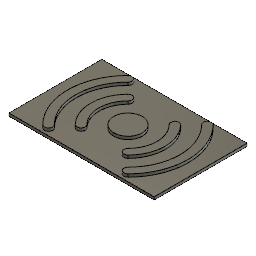
Glas (Autodesk Fusion 360 design; units mm, degrees)
Autodesk Fusion 360 part; units mm, degrees
sketch "Skizze1" plane through (0, 0, 0) normal (0, 1, 0) x (1, 0, 0)
  line L0 (25, 16) -> (-25, 16)
  line L1 (-25, 16) -> (-25, -16)
  line L2 (-25, -16) -> (25, -16)
  line L3 (25, -16) -> (25, 16)
  line L4 (25, 16) -> (-25, -16) construction
  line L5 (-25, 16) -> (25, -16) construction
  dimension "d1" = 50
  dimension "d2" = 32
  constraint horizontal L0
  constraint perpendicular L0 L1
  constraint parallel L0 L2
  constraint parallel L1 L3
  measures "d1" distance of L1.end L2.end
  measures "d2" distance of L0.end L1.end
extrude "Extrusion1" add sketch "Skizze1" along normal blind 1
sketch "Skizze2" plane through (0, 1, 0) normal (0, 1, 0) x (-1, 0, 0)
  line L0 (-25, 16) -> (-25, -16)
  line L1 (-25, -16) -> (25, -16)
  line L2 (25, -16) -> (25, 16)
  line L3 (25, 16) -> (-25, 16)
  circle A0 centre (0, 0) radius 4.9
  line L4 (0, 0) -> (0, -16) construction
  line L5 (0, 0) -> (-14.6371, -14.6371) construction
  line L6 (0, 0) -> (-14.6371, 14.6371) construction
  arc A1 (-7.0711, 7.0711) -> (-9.051, 9.051) centre (-8.061, 8.061) ccw
  arc A2 (-12.6572, 12.6572) -> (-14.6371, 14.6371) centre (-13.6472, 13.6472) ccw
  arc A3 (-9.051, 9.051) -> (-9.051, -9.051) centre (0, 0) ccw
  arc A4 (-7.0711, 7.0711) -> (-7.0711, -7.0711) centre (0, 0) ccw
  arc A5 (-14.6371, -14.6371) -> (-12.6572, -12.6572) centre (-13.6472, -13.6472) ccw
  arc A6 (-9.051, -9.051) -> (-7.0711, -7.0711) centre (-8.061, -8.061) ccw
  arc A7 (-12.6572, 12.6572) -> (-12.6572, -12.6572) centre (0, 0) ccw
  arc A8 (-14.6371, 14.6371) -> (-14.6371, -14.6371) centre (0, 0) ccw
  arc A9 (12.6572, -12.6572) -> (12.6572, 12.6572) centre (0, 0) ccw
  arc A10 (14.6371, -14.6371) -> (14.6371, 14.6371) centre (0, 0) ccw
  line L7 (25, 16) -> (25, -16)
  line L8 (0, 0) -> (14.6371, 14.6371) construction
  line L9 (25, -16) -> (-25, -16)
  arc A11 (9.051, -9.051) -> (9.051, 9.051) centre (0, 0) ccw
  arc A12 (12.6572, -12.6572) -> (14.6371, -14.6371) centre (13.6472, -13.6472) ccw
  arc A13 (7.0711, -7.0711) -> (7.0711, 7.0711) centre (0, 0) ccw
  line L10 (0, 0) -> (14.6371, -14.6371) construction
  arc A14 (9.051, 9.051) -> (7.0711, 7.0711) centre (8.061, 8.061) ccw
  line L11 (-25, 16) -> (25, 16)
  arc A15 (7.0711, -7.0711) -> (9.051, -9.051) centre (8.061, -8.061) ccw
  arc A16 (14.6371, 14.6371) -> (12.6572, 12.6572) centre (13.6472, 13.6472) ccw
  dimension "d6" = 9.8
  dimension "d7" = 2.8
  dimension "d8" = 5.1
  dimension "d9" = 5.1
  dimension "d10" = 2.8
  dimension "d11" = 45
  constraint coincident A0.centre L4.start
  constraint concentric A0 A3
  constraint concentric A0 A8
  constraint midpoint L1 L4.end
  constraint perpendicular L5 L6
  constraint coincident L5 A6.centre
  constraint coincident L5 A5.centre
  constraint tangent A3 A6
  constraint tangent A4 A6
  constraint tangent A5 A7
  constraint tangent A5 A8
  constraint tangent A2 A7
  constraint tangent A2 A8
  constraint coincident L6 A2.centre
  constraint coincident L6 A1.centre
  constraint tangent A1 A3
  constraint tangent A1 A4
  constraint coincident L5 A3.end
  constraint coincident L5 A4.end
  constraint coincident L5 A5.end
  constraint symmetric L0.start L4 L2.end
  constraint symmetric L0.end L4 L1.end
  constraint symmetric L1.end L4 L0.end
  constraint symmetric L2.end L4 L0.start
  constraint symmetric L4 A0.centre L5.start
  constraint symmetric L4 L5.end A10.start
  constraint symmetric L4 L6.end A10.end
  constraint symmetric L4 A1.end A11.end
  constraint symmetric L4 A1.start A13.end
  constraint symmetric L4 A1 A14
  constraint symmetric L4 A2.start A9.end
  constraint symmetric L4 A2 A16
  constraint symmetric L4 A3 A11
  constraint symmetric L4 A4 A13
  constraint symmetric L4 A3.end A11.start
  constraint symmetric L4 A4.end A13.start
  constraint symmetric L4 A5.end A9.start
  constraint symmetric L4 A5 A12
  constraint symmetric L4 A6 A15
  constraint symmetric L4 A7 A9
  constraint symmetric L4 A8 A10
  measures "d6" diameter of A0
  measures "d7" distance of A3 A4
  measures "d8" distance of A0 A4
  measures "d9" distance of A3 A7
  measures "d10" distance of A7 A8
  measures "d11" angle of L4 L5
extrude "Extrusion2" add sketch "Skizze2" along normal blind 1 contours A0 | A1 A3 A4 A6 | A2 A5 A7 A8 | A9 A10 A12 A16 | A11 A13 A14 A15
equation "d9 = d8"
equation "d10 = d7"
